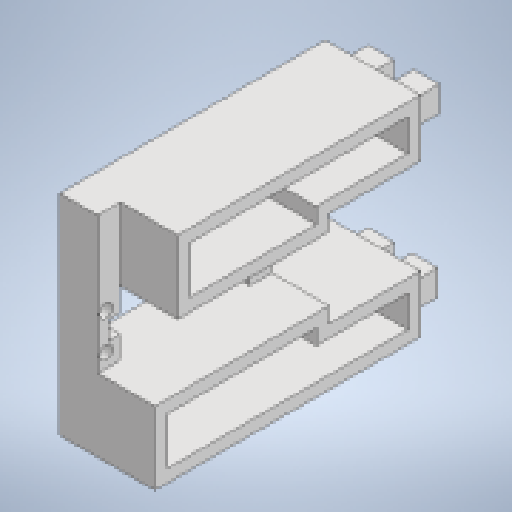
# Autodesk Inventor part: Adaptador servo
Saved by Autodesk Inventor 2024 (Build 280153000, 153)
## iProperties
Created: 2025-03-02
Part Number: Adaptador servo
Material: Genérico
Document SubType Name: Modeling
Designer: sergi
Density: 1 g/cm^3
Appearance: Valor por defecto
Author: sergi
Autodesk Inventor part; units mm, degrees
ref_plane "YZ Plane" through (0, 0, 0) normal (1, 0, 0) x (0, 1, 0)
ref_plane "XZ Plane" through (0, 0, 0) normal (0, 1, 0) x (-1, 0, 0)
ref_plane "XY Plane" through (0, 0, 0) normal (0, 0, 1) x (1, 0, 0)
ref_plane "Plano de trabajo1" through (30, -18, -46) normal (1, 0, 0) x (0, 1, 0)
sketch "Boceto1" plane through (0, 0, 0) normal (1, 0, 0) x (0, 1, 0)
  line L0 (-18, 0) -> (48, 0)
  line L1 (48, 0) -> (48, -11)
  line L2 (48, -11) -> (38, -11)
  line L3 (38, -11) -> (38, -46)
  line L4 (38, -46) -> (-8, -46)
  line L5 (-8, -46) -> (-8, -11)
  line L6 (-8, -11) -> (-18, -11)
  line L7 (-18, -11) -> (-18, 0)
  line L8 (5.1, 76.5) -> (5.1, 36)
  line L9 (5.1, 36) -> (24.9, 36)
  line L10 (24.9, 76.5) -> (24.9, 36)
  line L11 (5.1, 76.5) -> (24.9, 76.5)
  line L12 (5.1, 76.5) -> (24.9, 76.5)
  line L13 (-18, 0) -> (48, 0)
  line L14 (15.5, 83.65) -> (22.9, 83.65)
  line L15 (7.1, 83.65) -> (14.5, 83.65)
  line L16 (24.9, 76.5) -> (24.9, 36)
  line L17 (7.1, 83.65) -> (22.9, 83.65)
  line L18 (-18, 0) -> (48, 0)
  line L19 (48, 0) -> (48, 83.65)
  line L20 (48, 83.65) -> (-18, 83.65)
  line L21 (-18, 83.65) -> (-18, 0)
  line L22 (5.1, 76.5) -> (24.9, 76.5)
  line L23 (24.9, 76.5) -> (24.9, 0)
  line L24 (24.9, 0) -> (5.1, 0)
  line L25 (5.1, 0) -> (5.1, 76.5)
  line L26 (4.9, 76.7) -> (25.1, 76.7)
  line L27 (25.1, 76.7) -> (25.1, -0.2)
  line L28 (25.1, -0.2) -> (4.9, -0.2)
  line L29 (4.9, -0.2) -> (4.9, 76.7)
  line L30 (25.1, 0) -> (30, 0)
  line L31 (30, 0) -> (0, 0)
  line L32 (7.1, 28.85) -> (14.5, 28.85)
  line L33 (15.5, 28.85) -> (22.9, 28.85)
  line L34 (0, 0) -> (30, 0)
  line L35 (30, 0) -> (30, 28.85)
  line L36 (30, 28.85) -> (0, 28.85)
  line L37 (0, 28.85) -> (0, 0)
  line L38 (5.1, 36) -> (4.9, 36)
  line L39 (24.9, 36) -> (25.1, 36)
  line L40 (25.1, 35.8) -> (4.9, 35.8)
  line L41 (4.9, 35.8) -> (4.9, 76.5)
  point P0 (4.9, 0)
  point P1 (4.9, 28.85)
  point P2 (25.1, 28.85)
  point P3 (4.9, 35.8)
extrude "Extrusión1" add sketch "Boceto1" along normal up to surface (30 mm away) contours L21 L20 L15 L17 L14 L19 L0 L35 L36 L27 L26 L29 L37 | L29 L40 L25 L36 | L25 L40 L23 L36 L33 L32 | L23 L40 L27 L36
sketch "Boceto2" plane through (0, -18, 83.65) normal (0, 0, 1) x (1, 0, 0)
  line L0 (30, 43.1) -> (30, 22.9) projected
  line L1 (0, 22.9) -> (30, 22.9) projected
  line L2 (0, 22.9) -> (0, 43.1) projected
  line L3 (0, 43.1) -> (30, 43.1) projected
  line L4 (0, 66) -> (30, 66) projected
  line L5 (30, 22.9) -> (12, 22.9)
  line L6 (12, 22.9) -> (12, 66)
  line L7 (12, 66) -> (30, 66)
  line L8 (30, 66) -> (30, 22.9)
  point P0 (0, 18)
  dimension "d6" = 18
  constraints: 8 end point, 2 parallel, 1 horizontal, 1 perpendicular, 1 point on line
  measures "d6" distance of L6.end L7.end
ref_plane "Plano de trabajo2" through (0, 5.1, 76.5) normal (0, 0, 1) x (1, 0, 0)
extrude "Extrusión2" cut sketch "Boceto2" against normal up to surface (7.15 mm away) contours L0 L1 L6 L3 | L3 L6 L4 L8
sketch "Boceto3" plane through (0, -18, 0) normal (0, 0, -1) x (-1, 0, 0)
  line L0 (-26, 4) -> (-17.8, 4) projected
  line L1 (-26, 12.2) -> (-26, 4) projected
  line L2 (-17.8, 12.2) -> (-26, 12.2) projected
  line L3 (-17.8, 4) -> (-17.8, 12.2) projected
  line L4 (-4, 12.2) -> (-12.2, 12.2) projected
  line L5 (-4, 4) -> (-4, 12.2) projected
  line L6 (-12.2, 4) -> (-4, 4) projected
  line L7 (-12.2, 12.2) -> (-12.2, 4) projected
  line L8 (-26, 53.8) -> (-17.8, 53.8) projected
  line L9 (-26, 62) -> (-26, 53.8) projected
  line L10 (-17.8, 62) -> (-26, 62) projected
  line L11 (-17.8, 53.8) -> (-17.8, 62) projected
  line L12 (-4, 62) -> (-12.2, 62) projected
  line L13 (-4, 53.8) -> (-4, 62) projected
  line L14 (-12.2, 53.8) -> (-4, 53.8) projected
  line L15 (-12.2, 62) -> (-12.2, 53.8) projected
  line L16 (-4.1, 12.1) -> (-12.1, 12.1)
  line L17 (-12.1, 12.1) -> (-12.1, 4.1)
  line L18 (-12.1, 4.1) -> (-4.1, 4.1)
  line L19 (-4.1, 4.1) -> (-4.1, 12.1)
  line L20 (-17.9, 12.1) -> (-25.9, 12.1)
  line L21 (-25.9, 12.1) -> (-25.9, 4.1)
  line L22 (-25.9, 4.1) -> (-17.9, 4.1)
  line L23 (-17.9, 4.1) -> (-17.9, 12.1)
  line L24 (-17.9, 53.9) -> (-25.9, 53.9)
  line L25 (-25.9, 53.9) -> (-25.9, 61.9)
  line L26 (-25.9, 61.9) -> (-17.9, 61.9)
  line L27 (-17.9, 61.9) -> (-17.9, 53.9)
  line L28 (-4.1, 53.9) -> (-4.1, 61.9)
  line L29 (-4.1, 61.9) -> (-12.1, 61.9)
  line L30 (-12.1, 61.9) -> (-12.1, 53.9)
  line L31 (-12.1, 53.9) -> (-4.1, 53.9)
  point P0 (0, 18)
  dimension "d9" = 0.1
  dimension "d10" = 0.1
  dimension "d11" = 0.1
  dimension "d12" = 0.1
  constraints: 32 end point, 12 other
  measures "d9" distance between parallel lines of L5 L19
  measures "d10" distance between parallel lines of L3 L23
  measures "d11" distance between parallel lines of L8 L24
  measures "d12" distance between parallel lines of L14 L31
extrude "Extrusión3" add sketch "Boceto3" along normal blind 10 contours L19 L18 L17 L16 | L23 L22 L21 L20 | L24 L25 L26 L27 | L31 L30 L29 L28
chamfer "Chaflán1" distance 0.5 angle 45 12 edges at (4.1, 39.9, -10) (8.1, 35.9, -10) (8.1, 43.9, -10) (12.1, 39.9, -10) (4.1, -9.9, -10) (8.1, -5.9, -10) (8.1, -13.9, -10) (12.1, -9.9, -10) (17.9, -9.9, -10) (21.9, -5.9, -10) (21.9, -13.9, -10) (25.9, -9.9, -10)
sketch "Boceto4" plane through (12, 4.9, 83.65) normal (1, 0, 0) x (0, 0, -1)
  circle A0 centre (2.55, 15.8) radius 2.2 projected
  circle A1 centre (2.55, 4.4) radius 2.2 projected
  line L0 (7.15, 13) -> (7.15, 7.2) projected
  line L1 (7.15, 13) -> (3.25, 13) projected
  line L2 (3.25, 7.2) -> (3.25, 13) projected
  line L3 (7.15, 7.2) -> (3.25, 7.2) projected
  point P0 (83.65, -4.9)
extrude "Extrusión4" cut sketch "Boceto4" against normal through all contours L0 L3 L2 L1
sketch "Boceto7" plane through (0, 4.9, 35.8) normal (0, 0, 1) x (1, 0, 0)
  line L0 (12, 0) -> (12, 43.1) projected
  line L1 (0, 43.1) -> (12, 43.1) projected
  line L2 (0, 43.1) -> (0, -22.9) projected
  line L3 (0, -22.9) -> (30, -22.9) projected
  line L4 (30, -22.9) -> (30, 0) projected
  line L5 (30, 0) -> (12, 0) projected
  line L6 (30, 0) -> (30, 20.2) projected
  line L7 (0, 20.2) -> (30, 20.2) projected
  line L8 (0, 20.2) -> (0, 0) projected
  line L9 (0, 0) -> (30, 0) projected
  point P0 (0, -4.9)
  point P1 (12, 20.2)
extrude "Extrusión5" cut sketch "Boceto7" against normal through all contours L0 L7 L6 L5
sketch "Boceto5" plane through (12, 4.9, 83.65) normal (1, 0, 0) x (0, 0, -1)
  circle A0 centre (2.55, 15.8) radius 2.2 projected
  circle A1 centre (2.55, 4.4) radius 2.2 projected
  circle A2 centre (2.55, 15.8) radius 2.1
  circle A3 centre (2.55, 4.4) radius 2.1
  circle A4 centre (52.25, 4.4) radius 2.2 projected
  circle A5 centre (52.25, 15.8) radius 2.2 projected
  point P0 (83.65, -4.9)
  dimension "d22" = 4.2
  dimension "d23" = 4.2
  constraints: 2 centre point, 2 coincident
  measures "d22" diameter of A2
  measures "d23" diameter of A3
hole "Agujero1" at (12, 9.3, 81.1) at (12, 20.7, 81.1) at (12, 9.3, 31.4) at (12, 20.7, 31.4) direction (-1, 0, 0) diameter 4.2 depth 5
sketch "Boceto6" plane through (7, 9.3, 81.1) normal (1, 0, 0) x (0, 0, -1)
  circle A0 centre (0, 11.4) radius 2.1 projected
  circle A1 centre (0, 0) radius 2.1 projected
  circle A2 centre (49.7, 0) radius 2.1 projected
  circle A3 centre (49.7, 11.4) radius 2.1 projected
  point P0 (81.1, -9.3)
  point P1 (0, 11.4)
  constraints: 4 coincident
hole "Agujero2" at (7, 20.7, 81.1) at (7, 9.3, 81.1) at (7, 9.3, 31.4) at (7, 20.7, 31.4) direction (-1, 0, 0) diameter 3.2 end through all
sketch "Boceto8" plane through (0, -18, 0) normal (0, -1, 0) x (1, 0, 0)
  circle A0 centre (5, 57) radius 1.6 projected
  circle A1 centre (5, 5) radius 1.6 projected
  point P0 (0, 0)
  point P1 (7.089064, 68.764863)
hole "Agujero3" at (5, -18, 57) at (5, -18, 5) direction (0, 1, 0) diameter 4.2 depth 5
sketch "Boceto9" plane through (0, 48, 83.65) normal (0, 1, 0) x (1, 0, 0)
  circle A0 centre (5, 26.65) radius 2.1 projected
  circle A1 centre (5, 78.65) radius 2.1 projected
  point P0 (0, 83.65)
hole "Agujero4" at (5, 48, 57) at (5, 48, 5) direction (0, -1, 0) diameter 4.2 depth 5
shell "Vaciado1" thickness 3.99999 removed faces 2 at (30, -12, 37.5) at (30, 42, 35.116667)
